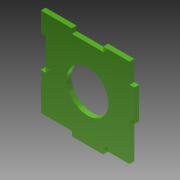
# Autodesk Inventor part: Side B
Saved by Autodesk Inventor 2014 SP2 (Build 180246200, 246)
## iProperties
Created: 2014-11-21
Part Number: Side B
Material: Generic
Document SubType Name: Modeling
Designer: JLM
Density: 1 g/cm^3
Appearance: Default
Author: JLM
Autodesk Inventor part; units mm, degrees
ref_plane "YZ Plane" through (0, 0, 0) normal (1, 0, 0) x (0, 1, 0)
ref_plane "XZ Plane" through (0, 0, 0) normal (0, 1, 0) x (-1, 0, 0)
ref_plane "XY Plane" through (0, 0, 0) normal (0, 0, 1) x (1, 0, 0)
sketch "Sketch1" plane through (0, 0, 0) normal (0, 0, 1) x (1, 0, 0)
  line L0 (-28.321, -28.321) -> (28.321, -28.321)
  line L1 (28.321, -28.321) -> (28.321, 28.321)
  line L2 (28.321, 28.321) -> (-28.321, 28.321)
  line L3 (-28.321, 28.321) -> (-28.321, -28.321)
  line L4 (-28.321, -28.321) -> (28.321, 28.321) construction
  line L5 (28.321, -28.321) -> (-28.321, 28.321) construction
  point P0 (0, 0)
  dimension "d0" = 56.642
  dimension "d1" = 56.642
  constraints: 12 end point, 2 midpoint, 2 parallel, 1 horizontal, 1 perpendicular
  measures "d0" distance of L2.end L1.end
  measures "d1" distance of L1.end L0.end
extrude "Extrusion1" add sketch "Sketch1" against normal blind 2.921
sketch "Sketch4" plane through (0, 0, 0) normal (0, 0, 1) x (1, 0, 0)
  line L0 (28.321, -25.4) -> (9.525, -25.4)
  line L1 (9.525, -25.4) -> (9.525, -28.321)
  line L2 (9.525, -28.321) -> (28.321, -28.321)
  line L3 (28.321, -28.321) -> (28.321, -25.4)
  line L4 (-28.321, -28.321) -> (-9.525, -28.321)
  line L5 (-9.525, -28.321) -> (-9.525, -25.4)
  line L6 (-9.525, -25.4) -> (-28.321, -25.4)
  line L7 (-28.321, -25.4) -> (-28.321, -28.321)
  line L8 (28.321, -28.321) -> (28.321, 28.321) projected
  line L9 (28.321, 28.321) -> (-28.321, 28.321) projected
  line L10 (-28.321, 28.321) -> (-28.321, -28.321) projected
  line L11 (-28.321, 16.129) -> (-25.4, 16.129)
  line L12 (-25.4, 16.129) -> (-25.4, -2.921)
  line L13 (-25.4, -2.921) -> (-28.321, -2.921)
  line L14 (-28.321, -2.921) -> (-28.321, 16.129)
  line L15 (28.321, 16.129) -> (25.4, 16.129)
  line L16 (25.4, 16.129) -> (25.4, -2.921)
  line L17 (25.4, -2.921) -> (28.321, -2.921)
  line L18 (28.321, -2.921) -> (28.321, 16.129)
  line L19 (-9.525, 28.321) -> (9.525, 28.321)
  line L20 (9.525, 28.321) -> (9.525, 25.4)
  line L21 (9.525, 25.4) -> (-9.525, 25.4)
  line L22 (-9.525, 25.4) -> (-9.525, 28.321)
  line L23 (-28.321, -28.321) -> (28.321, -28.321) projected
  line L24 (25.4, -2.921) -> (25.4, -28.321)
  line L25 (25.4, 16.129) -> (25.4, 28.321)
  point P0 (0, 0)
  dimension "d12" = 18.796
  dimension "d13" = 2.921
  dimension "d16" = 2.921
  dimension "d37" = 9.525
  dimension "d38" = 18.796
  dimension "d39" = 9.525
  dimension "d40" = 2.921
  dimension "d41" = 2.921
  dimension "d42" = 19.05
  dimension "d43" = 19.05
  dimension "d44" = 2.921
  dimension "d45" = 19.05
  dimension "d46" = 18.796
  dimension "d50" = 25.4
  dimension "d51" = 25.4
  dimension "d52" = 19.05
  dimension "d53" = 56.642
  dimension "d54" = 56.642
  constraints: 44 end point, 10 parallel, 7 perpendicular, 5 horizontal, 5 point on line, 2 collinear
  measures "d12" distance of L2.end L1.end
  measures "d13" distance of L1.end L0.end
  measures "d16" distance of L4.end L5.end
  measures "d37" distance from line of point (0, 0) L5
  measures "d38" distance of L4.start L4.end
  measures "d39" distance from line of point (0, 0) L1
  measures "d40" distance of L11.start L11.end
  measures "d41" distance of L15.start L15.end
  measures "d42" distance of L11.end L12.end
  measures "d43" distance of L15.end L16.end
  measures "d44" distance of L21.end L19.start
  measures "d45" distance of L20.end L21.end
  measures "d46" distance between parallel lines of L10 L22
  measures "d50" distance between parallel lines of L4 L13
  measures "d51" distance between parallel lines of L23 L17
  measures "d52" distance between parallel lines of L1 L5
  measures "d53" distance between parallel lines of L23 L9
  measures "d54" distance between parallel lines of L8 L10
extrude "Extrusion5" cut sketch "Sketch4" against normal blind 25.4 contours L3 L2 L24 L0 | L0 L24 L17 L8 | L24 L2 L1 L0 | L15 L25 L9 L8 | L4 L7 L6 L5 | L20 L21 L22 L9 | L10 L11 L12 L13
hole "Hole1" at (0, 0, 0) direction (0, 0, -1) diameter 25.4 end through all
equation "\"d1\" = d0"
equation "\"d12\" = d38"
equation "\"d13\" = d16"
equation "\"d38\" = -d37 + 0.5 * d0"
equation "\"d39\" = d37"
equation "\"d40\" = d16"
equation "\"d41\" = d16"
equation "\"d42\" = 2 * d37"
equation "\"d43\" = d42"
equation "\"d44\" = d16"
equation "\"d45\" = d42"
equation "\"d46\" = d38"
equation "\"d51\" = d50"
equation "\"d19\" = 0.5 * d0"
equation "\"d48\" = 0.5 * d0"
body "Solid1"
